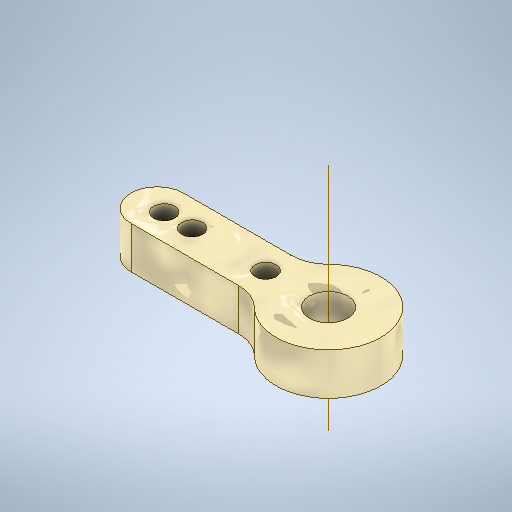
# Autodesk Inventor part: adaptator_25
Saved by Autodesk Inventor 2025 (Build 290162000, 162)
## iProperties
Created: 2024-12-10
Part Number: adaptator_25
Material: Generic
Document SubType Name: Modeling
Designer: Pauline Simonnet
Density: 1 g/cm^3
Appearance: Fine - Cream
Author: Pauline Simonnet
Autodesk Inventor part; units mm, degrees
ref_plane "YZ Plane" through (0, 0, 0) normal (1, 0, 0) x (0, 1, 0)
ref_plane "XZ Plane" through (0, 0, 0) normal (0, 1, 0) x (-1, 0, 0)
ref_plane "XY Plane" through (0, 0, 0) normal (0, 0, 1) x (1, 0, 0)
sketch "Sketch1" plane through (0, 0, 0) normal (0, 1, 0) x (-1, 0, 0)
  arc A0 (5.2699, 5.3365) -> (5.2699, -5.3365) centre (0, 0) ccw
  arc A1 (24.5, -3.75) -> (24.5, 3.75) centre (24.5, 0) ccw
  arc A2 (5.2699, 5.3365) -> (9.1344, 3.75) centre (9.1344, 9.25) ccw
  arc A3 (9.1344, -3.75) -> (5.2699, -5.3365) centre (9.1344, -9.25) ccw
  line L0 (9.1344, 3.75) -> (24.5, 3.75)
  line L1 (9.1344, -3.75) -> (24.5, -3.75)
  line L2 (0, 0) -> (39, 0) construction
  circle A4 centre (0, 0) radius 2.75
  circle A5 centre (9, 0) radius 1.5
  circle A6 centre (23.5, 0) radius 1.5
  circle A7 centre (19.5, 0) radius 1.5
  dimension "d0" = 15
  dimension "d1" = 7.5
  dimension "d2" = 24.5
  dimension "d3" = 7.5
  dimension "d4" = 11
  dimension "d5" = 11
  dimension "d6" = 0
  dimension "d7" = 3.75
  dimension "d8" = 5.5
  dimension "d9" = 3
  dimension "d10" = 3
  dimension "d11" = 3
  dimension "d12" = 9
  dimension "d13" = 10.5
  dimension "d14" = 4
  constraints: 8 centre point, 8 point on circle, 6 end point, 4 tangent, 3 horizontal, 2 coincident, 2 point on line, 1 midpoint
  measures "d0" diameter of A0
  measures "d1" diameter of A1
  measures "d2" distance of point (0, 0) A1.centre
  measures "d3" distance between parallel lines of L1 L0
  measures "d4" diameter of A2
  measures "d5" diameter of A3
  measures "d6" distance from line of L2 A1.centre
  measures "d7" distance between parallel lines of L2 L0
  measures "d8" diameter of A4
  measures "d9" diameter of A5
  measures "d10" diameter of A7
  measures "d11" diameter of A6
  measures "d12" distance of point (0, 0) A5.centre
  measures "d13" distance of A5.centre A7.centre
  measures "d14" distance of A7.centre A6.centre
extrude "Extrusion1" add sketch "Sketch1" along normal blind 6
equation "\"d5\" = d4"
body "Solid1"
